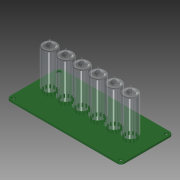
# Autodesk Inventor part: PCB3
Saved by Autodesk Inventor 2015 (Build 190159000, 159)
## iProperties
Created: 2018-03-01
Part Number: PCB3
Material: Generic
Document SubType Name: Modeling
Designer: Silas
Density: 1 g/cm^3
Appearance: Default
Author: Silas
Autodesk Inventor part; units mm, degrees
ref_plane "YZ Plane" through (0, 0, 0) normal (1, 0, 0) x (0, 1, 0)
ref_plane "XZ Plane" through (0, 0, 0) normal (0, 1, 0) x (-1, 0, 0)
ref_plane "XY Plane" through (0, 0, 0) normal (0, 0, 1) x (1, 0, 0)
sketch "Sketch1" plane through (0, 0, 0) normal (0, 0, 1) x (1, 0, 0)
  line L0 (0, 0) -> (99, 0)
  line L1 (99, 0) -> (99, 45.4)
  line L2 (99, 45.4) -> (0, 45.4)
  line L3 (0, 45.4) -> (0, 0)
  circle A0 centre (3, 42.4) radius 1.5
  circle A1 centre (3, 3) radius 1.5
  circle A2 centre (96, 3) radius 1.5
  circle A3 centre (96, 42.4) radius 1.5
  dimension "d0" = 45.4
  dimension "d1" = 99
  dimension "d2" = 3
  dimension "d3" = 3
  dimension "d4" = 3
  dimension "d5" = 3
  dimension "d6" = 3
  dimension "d7" = 3
  dimension "d8" = 3
  dimension "d9" = 3
  dimension "d10" = 3
  dimension "d11" = 3
  dimension "d12" = 3
  dimension "d13" = 3
  constraints: 8 end point, 4 centre point, 2 parallel, 1 horizontal, 1 perpendicular
  measures "d0" distance of L1.end L0.end
  measures "d1" distance of L1.end L2.end
  measures "d2" diameter of A0
  measures "d3" diameter of A1
  measures "d4" diameter of A2
  measures "d5" diameter of A3
  measures "d6" distance from line of L3 A0.centre
  measures "d7" distance from line of L2 A0.centre
  measures "d8" distance from line of L3 A1.centre
  measures "d9" distance from line of L0 A1.centre
  measures "d10" distance from line of L0 A2.centre
  measures "d11" distance from line of L1 A2.centre
  measures "d12" distance from line of L2 A3.centre
  measures "d13" distance from line of L1 A3.centre
extrude "Extrusion1" add sketch "Sketch1" along normal blind 1.6
fillet "Fillet1" radius 3 4 edges at (0, 0, 0.8) (99, 0, 0.8) (99, 45.4, 0.8) (0, 45.4, 0.8)
sketch "Sketch2" plane through (0, 0, 1.6) normal (0, 0, 1) x (1, 0, 0)
  circle A0 centre (14.5, 22.7) radius 6
  line L0 (0, 42.4) -> (0, 3) construction
  line L1 (0, 22.7) -> (99, 22.7) construction
  line L2 (99, 3) -> (99, 42.4) construction
  circle A1 centre (28.5, 22.7) radius 6
  circle A2 centre (42.5, 22.7) radius 6
  circle A3 centre (56.5, 22.7) radius 6
  circle A4 centre (70.5, 22.7) radius 6
  circle A5 centre (84.5, 22.7) radius 6
  point P0 (0, 0)
  dimension "d17" = 12
  dimension "d18" = 12
  dimension "d19" = 12
  dimension "d20" = 12
  dimension "d21" = 12
  dimension "d22" = 12
  dimension "d23" = 14
  dimension "d24" = 14
  dimension "d25" = 14
  dimension "d26" = 14
  dimension "d27" = 14
  dimension "d28" = 14.5
  dimension "d29" = 14.5
  constraints: 6 centre point, 6 point on line, 2 end point, 2 midpoint
  measures "d17" diameter of A0
  measures "d18" diameter of A1
  measures "d19" diameter of A2
  measures "d20" diameter of A3
  measures "d21" diameter of A4
  measures "d22" diameter of A5
  measures "d23" distance of A1.centre A0.centre
  measures "d24" distance of A2.centre A1.centre
  measures "d25" distance of A3.centre A2.centre
  measures "d26" distance of A4.centre A3.centre
  measures "d27" distance of A5.centre A4.centre
  measures "d28" distance of L1.start A0.centre
  measures "d29" distance of L1.end A5.centre
extrude "Extrusion2" add sketch "Sketch2" along normal blind 35
sketch "Sketch3" plane through (14.5, 22.7, 36.6) normal (0, 0, 1) x (1, 0, 0)
  circle A0 centre (0, 0) radius 6 construction
  circle A1 centre (14, 0) radius 6 construction
  circle A2 centre (28, 0) radius 6 construction
  circle A3 centre (42, 0) radius 6 construction
  circle A4 centre (56, 0) radius 6 construction
  circle A5 centre (70, 0) radius 6 construction
  circle A6 centre (70, 0) radius 0.5
  circle A7 centre (56, 0) radius 0.5
  circle A8 centre (42, 0) radius 0.5
  circle A9 centre (28, 0) radius 0.5
  circle A10 centre (14, 0) radius 0.5
  circle A11 centre (0, 0) radius 0.5
  point P0 (-14.5, -22.7)
  dimension "d32" = 1
  dimension "d33" = 1
  dimension "d34" = 1
  dimension "d35" = 1
  dimension "d36" = 1
  dimension "d37" = 1
  constraints: 6 centre point, 6 coincident
  measures "d32" diameter of A6
  measures "d33" diameter of A7
  measures "d34" diameter of A8
  measures "d35" diameter of A9
  measures "d36" diameter of A10
  measures "d37" diameter of A11
extrude "Extrusion3" add sketch "Sketch3" along normal blind 5
fillet "Fillet2" radius 5 6 edges at (14, 22.7, 36.6) (28, 22.7, 36.6) (42, 22.7, 36.6) (56, 22.7, 36.6) (70, 22.7, 36.6) (84, 22.7, 36.6)
fillet "Fillet3" radius 0.5 12 edges at (14, 22.7, 41.5995) (14, 22.7, 41.6) (28, 22.7, 41.5995) (28, 22.7, 41.6) (42, 22.7, 41.5995) (42, 22.7, 41.6) (56, 22.7, 41.5995) (56, 22.7, 41.6) (70, 22.7, 41.5995) (70, 22.7, 41.6) (84, 22.7, 41.5995) (84, 22.7, 41.6)
sketch "Sketch4" plane through (0, 0, 1.6) normal (0, 0, 1) x (1, 0, 0)
  circle A0 centre (84.5, 22.7) radius 6 projected
  circle A1 centre (70.5, 22.7) radius 6 projected
  circle A2 centre (56.5, 22.7) radius 6 projected
  circle A3 centre (42.5, 22.7) radius 6 projected
  circle A4 centre (28.5, 22.7) radius 6 projected
  circle A5 centre (14.5, 22.7) radius 6 projected
  circle A6 centre (19, 22.7) radius 0.5
  line L0 (14.5, 22.7) -> (20.5, 22.7) construction
  circle A7 centre (18.2856, 25.1329) radius 0.5
  circle A8 centre (16.3694, 26.7933) radius 0.5
  circle A9 centre (13.8596, 27.1542) radius 0.5
  circle A10 centre (11.5531, 26.1009) radius 0.5
  circle A11 centre (10.1823, 23.9678) radius 0.5
  circle A12 centre (10.1823, 21.4322) radius 0.5
  circle A13 centre (11.5531, 19.2991) radius 0.5
  circle A14 centre (13.8596, 18.2458) radius 0.5
  circle A15 centre (16.3694, 18.6067) radius 0.5
  circle A16 centre (18.2856, 20.2671) radius 0.5
  line L1 (28.5, 22.7) -> (22.5, 22.7) construction
  line L2 (22.5, 22.7) -> (20.5, 22.7) construction
  line L3 (21.5, 22.7) -> (21.5, 19.5758) construction
  circle A17 centre (24, 22.7) radius 0.5
  circle A18 centre (24.7144, 25.1329) radius 0.5
  circle A19 centre (26.6306, 26.7933) radius 0.5
  circle A20 centre (29.1404, 27.1542) radius 0.5
  circle A21 centre (31.4469, 26.1009) radius 0.5
  circle A22 centre (32.8177, 23.9678) radius 0.5
  circle A23 centre (32.8177, 21.4322) radius 0.5
  circle A24 centre (31.4469, 19.2991) radius 0.5
  circle A25 centre (29.1404, 18.2458) radius 0.5
  circle A26 centre (26.6306, 18.6067) radius 0.5
  circle A27 centre (24.7144, 20.2671) radius 0.5
  line L4 (34.5, 22.7) -> (36.5, 22.7) construction
  line L5 (35.5, 22.7) -> (35.5, 16.7) construction
  circle A28 centre (47, 22.7) radius 0.5
  circle A29 centre (46.2856, 25.1329) radius 0.5
  circle A30 centre (44.3694, 26.7933) radius 0.5
  circle A31 centre (41.8596, 27.1542) radius 0.5
  circle A32 centre (39.5531, 26.1009) radius 0.5
  circle A33 centre (46.2856, 20.2671) radius 0.5
  circle A34 centre (44.3694, 18.6067) radius 0.5
  circle A35 centre (41.8596, 18.2458) radius 0.5
  circle A36 centre (39.5531, 19.2991) radius 0.5
  circle A37 centre (38.1823, 21.4322) radius 0.5
  circle A38 centre (38.1823, 23.9678) radius 0.5
  line L6 (3, 0) -> (96, 0) construction
  line L7 (49.5, 0) -> (49.5, 45.4) construction
  line L8 (96, 45.4) -> (3, 45.4) construction
  circle A39 centre (80, 22.7) radius 0.5
  circle A40 centre (80.7144, 25.1329) radius 0.5
  circle A41 centre (82.6306, 26.7933) radius 0.5
  circle A42 centre (85.1404, 27.1542) radius 0.5
  circle A43 centre (87.4469, 26.1009) radius 0.5
  circle A44 centre (88.8177, 23.9678) radius 0.5
  circle A45 centre (88.8177, 21.4322) radius 0.5
  circle A46 centre (87.4469, 19.2991) radius 0.5
  circle A47 centre (85.1404, 18.2458) radius 0.5
  circle A48 centre (82.6306, 18.6067) radius 0.5
  circle A49 centre (80.7144, 20.2671) radius 0.5
  circle A50 centre (75, 22.7) radius 0.5
  circle A51 centre (74.2856, 25.1329) radius 0.5
  circle A52 centre (72.3694, 26.7933) radius 0.5
  circle A53 centre (69.8596, 27.1542) radius 0.5
  circle A54 centre (67.5531, 26.1009) radius 0.5
  circle A55 centre (74.2856, 20.2671) radius 0.5
  circle A56 centre (72.3694, 18.6067) radius 0.5
  circle A57 centre (69.8596, 18.2458) radius 0.5
  circle A58 centre (67.5531, 19.2991) radius 0.5
  circle A59 centre (66.1823, 21.4322) radius 0.5
  circle A60 centre (66.1823, 23.9678) radius 0.5
  circle A61 centre (59.4469, 19.2991) radius 0.5
  circle A62 centre (60.8177, 21.4322) radius 0.5
  circle A63 centre (60.8177, 23.9678) radius 0.5
  circle A64 centre (59.4469, 26.1009) radius 0.5
  circle A65 centre (57.1404, 27.1542) radius 0.5
  circle A66 centre (54.6306, 26.7933) radius 0.5
  circle A67 centre (52.7144, 25.1329) radius 0.5
  circle A68 centre (52, 22.7) radius 0.5
  circle A69 centre (52.7144, 20.2671) radius 0.5
  circle A70 centre (54.6306, 18.6067) radius 0.5
  circle A71 centre (57.1404, 18.2458) radius 0.5
  point P0 (0, 0)
  dimension "d43" = 1
  dimension "d44" = 4.5
  dimension "d47" = 360
  constraints: 66 centre point, 55 symmetric about line, 14 end point, 4 midpoint, 3 horizontal, 2 horizontal alignment, 2 point on circle, 2 vertical, 1 point on line, 80 other
  measures "d43" diameter of A6
  measures "d44" distance of L0.start A6.centre
extrude "Extrusion4" cut sketch "Sketch4" along normal blind 3
fillet "Fillet4" radius 1 12 edges at (8.5, 22.7, 36.6) (22.5, 22.7, 36.6) (36.5, 22.7, 36.6) (50.5, 22.7, 36.6) (64.5, 22.7, 36.6) (78.5, 22.7, 36.6) (8.5, 22.7, 4.6) (22.5, 22.7, 4.6) (36.5, 22.7, 4.6) (50.5, 22.7, 4.6) (64.5, 22.7, 4.6) (78.5, 22.7, 4.6)
equation "\"d7\" = d6"
equation "\"d8\" = d9"
equation "\"d9\" = d7"
equation "\"d10\" = d11"
equation "\"d11\" = d8"
equation "\"d12\" = d10"
equation "\"d13\" = d12"
equation "\"d24\" = d23"
equation "\"d25\" = d24"
equation "\"d26\" = d25"
equation "\"d27\" = d26"
equation "\"d28\" = d29"
body "Solid1"
